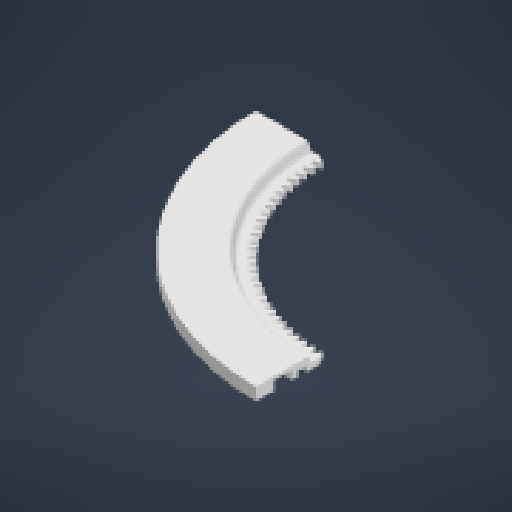
# Autodesk Inventor part: outerspinner_v3
Saved by Autodesk Inventor 2026 (Build 300175050, 175E)
## iProperties
Created: 2026-04-30
Part Number: outerspinner_v3
Material: Generic
Document SubType Name: Modeling
Designer: sniel
Density: 1 g/cm^3
Appearance: Default
Author: sniel
Autodesk Inventor part; units mm, degrees
(part 1 of 2)
ref_plane "YZ Plane" through (0, 0, 0) normal (1, 0, 0) x (0, 1, 0)
ref_plane "XZ Plane" through (0, 0, 0) normal (0, 1, 0) x (-1, 0, 0)
ref_plane "XY Plane" through (0, 0, 0) normal (0, 0, 1) x (1, 0, 0)
sketch "Sketch1" plane through (0, 0, 0) normal (1, 0, 0) x (0, 1, 0)
  line L0 (0, -11.1) -> (7, -11.1)
  line L1 (0, -122.2355) -> (0, -11.1)
  line L2 (13, -122.2355) -> (0, -122.2355)
  line L3 (13, -121.3855) -> (13, -122.2355)
  line L4 (8, -121.3855) -> (13, -121.3855)
  line L5 (8, -115.0855) -> (8, -121.3855)
  line L6 (13, -115.0855) -> (8, -115.0855)
  line L7 (13, -114.2355) -> (13, -115.0855)
  line L8 (7, -114.2355) -> (13, -114.2355)
  line L9 (7, -11.1) -> (7, -114.2355)
  line L10 (7, 11.1) -> (0, 11.1)
  line L11 (7, 114.2355) -> (7, 11.1)
  line L12 (13, 114.2355) -> (7, 114.2355)
  line L13 (13, 115.0855) -> (13, 114.2355)
  line L14 (8, 115.0855) -> (13, 115.0855)
  line L15 (8, 121.3855) -> (8, 115.0855)
  line L16 (13, 121.3855) -> (8, 121.3855)
  line L17 (13, 122.2355) -> (13, 121.3855)
  line L18 (0, 122.2355) -> (13, 122.2355)
  line L19 (0, 11.1) -> (0, 122.2355)
  line L20 (8, 118.2355) -> (13.9, 118.2355)
  line L21 (13.9, 118.2355) -> (13.9, 103.2355)
  line L22 (13.9, 118.2355) -> (13.9, 133.2355)
  line L23 (13.9, 133.2355) -> (15.9, 133.2355)
  line L24 (15.9, 133.2355) -> (15.9, 103.2355)
  line L25 (15.9, 103.2355) -> (13.9, 103.2355)
  line L26 (13.9, 118.2355) -> (13.9, 123.2355)
  line L27 (13.9, 123.2355) -> (8.9, 123.2355)
  line L28 (8.9, 123.2355) -> (8.9, 133.2355)
  line L29 (8.9, 133.2355) -> (13.9, 133.2355)
  line L30 (13.9, 118.2355) -> (13.9, 113.2355)
  line L31 (13.9, 113.2355) -> (8.9, 113.2355)
  line L32 (8.9, 113.2355) -> (8.9, 103.2355)
  line L33 (8.9, 103.2355) -> (13.9, 103.2355)
  line L34 (-3.18, 0) -> (19.08, 0) projected
  dimension "d0" = 5.9
  dimension "d1" = 15
  dimension "d2" = 15
  dimension "d3" = 2
  dimension "d4" = 5
  dimension "d5" = 5
  dimension "d6" = 5
  constraints: 68 end point, 7 perpendicular, 3 horizontal, 2 point on line, 2 vertical, 1 midpoint
  measures "d0" distance of L20.start L20.end
  measures "d1" distance of L20.end L21.end
  measures "d2" distance of L20.end L22.end
  measures "d3" distance of L22.end L23.end
  measures "d4" distance of L20.end L26.end
  measures "d5" distance of L26.end L27.end
  measures "d6" distance of L20.end L30.end
revolve "Revolution1" add sketch "Sketch1" angle 360 about axis through (0, -10, 0) along (0, 1, 0) contours L22 L23 L24 L25 L21 | L21 L33 L32 L31 | L27 L28 L29 L22
sketch "Sketch2" plane through (0, 0, 0) normal (1, 0, 0) x (0, 1, 0)
  line L0 (55, 175) -> (-32, 175)
  line L1 (-32, 175) -> (-32, -166)
  line L2 (-32, -166) -> (55, -166)
  line L3 (55, -166) -> (55, 175)
  point P0 (0, 0)
  constraints: 8 end point, 2 parallel, 1 horizontal, 1 perpendicular
extrude "Extrusion1" cut sketch "Sketch2" along normal blind 157.75
sketch "Sketch3" plane through (0, 8.9, 0) normal (0, -1, 0) x (1, 0, 0)
  arc A0 (-6.4389, -92.6782) -> (-5.913, -96.4432) centre (11.3389, -92.1143) ccw
  arc A1 (-5.913, -96.4432) -> (-4.6085, -96.6498) centre (0, -63.3314) ccw
  arc A2 (-4.6085, -96.6498) -> (-2.9449, -93.2316) centre (-19.6784, -87.2016) ccw
  arc A3 (-2.9449, -93.2316) -> (-1.7688, -93.3241) centre (0, -63.3314) ccw
  arc A4 (-1.7688, -93.3241) -> (-0.6604, -96.9605) centre (15.702, -89.9861) ccw
  arc A5 (-0.6604, -96.9605) -> (0.6604, -96.9605) centre (0, -63.3314) ccw
  arc A6 (0.6604, -96.9605) -> (1.7688, -93.3241) centre (-15.702, -89.9861) ccw
  arc A7 (1.7688, -93.3241) -> (2.9449, -93.2316) centre (0, -63.3314) ccw
  arc A8 (2.9449, -93.2316) -> (4.6085, -96.6498) centre (19.6784, -87.2016) ccw
  arc A9 (4.6085, -96.6498) -> (5.913, -96.4432) centre (0, -63.3314) ccw
  arc A10 (5.913, -96.4432) -> (6.4389, -92.6782) centre (-11.3389, -92.1143) ccw
  arc A11 (6.4389, -92.6782) -> (7.5861, -92.4028) centre (0, -63.3314) ccw
  arc A12 (7.5861, -92.4028) -> (9.7639, -95.5186) centre (23.1702, -83.8294) ccw
  arc A13 (9.7639, -95.5186) -> (11.02, -95.1105) centre (0, -63.3314) ccw
  arc A14 (11.02, -95.1105) -> (10.9505, -91.3096) centre (-6.6967, -93.5337) ccw
  arc A15 (10.9505, -91.3096) -> (12.0404, -90.8581) centre (0, -63.3314) ccw
  arc A16 (12.0404, -90.8581) -> (14.6789, -93.595) centre (26.0915, -79.9524) ccw
  arc A17 (14.6789, -93.595) -> (15.8557, -92.9953) centre (0, -63.3314) ccw
  arc A18 (15.8557, -92.9953) -> (15.1924, -89.2521) centre (-1.8896, -94.2095) ccw
  arc A19 (15.1924, -89.2521) -> (16.1983, -88.6357) centre (0, -63.3314) ccw
  arc A20 (16.1983, -88.6357) -> (19.2324, -90.9261) centre (28.3704, -75.6661) ccw
  arc A21 (19.2324, -90.9261) -> (20.3009, -90.1497) centre (0, -63.3314) ccw
  arc A22 (20.3009, -90.1497) -> (19.0602, -86.5564) centre (2.9641, -94.1249) ccw
  arc A23 (19.0602, -86.5564) -> (19.9574, -85.7902) centre (0, -63.3314) ccw
  arc A24 (19.9574, -85.7902) -> (23.3124, -87.5777) centre (29.9507, -71.0762) ccw
  arc A25 (23.3124, -87.5777) -> (24.2463, -86.6438) centre (0, -63.3314) ccw
  arc A26 (24.2463, -86.6438) -> (22.4588, -83.2888) centre (7.7447, -93.2821) ccw
  arc A27 (22.4588, -83.2888) -> (23.225, -82.3917) centre (0, -63.3314) ccw
  arc A28 (23.225, -82.3917) -> (26.8183, -83.6324) centre (30.7935, -66.2955) ccw
  arc A29 (26.8183, -83.6324) -> (27.5947, -82.5638) centre (0, -63.3314) ccw
  arc A30 (27.5947, -82.5638) -> (25.3043, -79.5297) centre (12.3347, -91.7018) ccw
  arc A31 (25.3043, -79.5297) -> (25.9207, -78.5238) centre (0, -63.3314) ccw
  arc A32 (25.9207, -78.5238) -> (29.6639, -79.1871) centre (30.878, -61.4418) ccw
  arc A33 (29.6639, -79.1871) -> (30.2635, -78.0103) centre (0, -63.3314) ccw
  arc A34 (30.2635, -78.0103) -> (27.5267, -75.3718) centre (16.621, -89.4229) ccw
  arc A35 (27.5267, -75.3718) -> (27.9782, -74.2819) centre (0, -63.3314) ccw
  arc A36 (27.9782, -74.2819) -> (31.7791, -74.3514) centre (30.2023, -56.6347) ccw
  arc A37 (31.7791, -74.3514) -> (32.1872, -73.0953) centre (0, -63.3314) ccw
  arc A38 (32.1872, -73.0953) -> (29.0714, -70.9175) centre (20.4979, -86.5016) ccw
  arc A39 (29.0714, -70.9175) -> (29.3468, -69.7703) centre (0, -63.3314) ccw
  arc A40 (29.3468, -69.7703) -> (33.1117, -69.2444) centre (28.7829, -51.9925) ccw
  arc A41 (33.1117, -69.2444) -> (33.3184, -67.9399) centre (0, -63.3314) ccw
  arc A42 (33.3184, -67.9399) -> (29.9002, -66.2763) centre (23.8702, -83.0098) ccw
  arc A43 (29.9002, -66.2763) -> (29.9927, -65.1002) centre (0, -63.3314) ccw
  arc A44 (29.9927, -65.1002) -> (33.6291, -63.9918) centre (26.6547, -47.6295) ccw
  arc A45 (33.6291, -63.9918) -> (33.6291, -62.671) centre (0, -63.3314) ccw
  arc A46 (33.6291, -62.671) -> (29.9927, -61.5627) centre (26.6547, -79.0334) ccw
  arc A47 (29.9927, -61.5627) -> (29.9002, -60.3865) centre (0, -63.3314) ccw
  arc A48 (29.9002, -60.3865) -> (33.3184, -58.7229) centre (23.8702, -43.6531) ccw
  arc A49 (33.3184, -58.7229) -> (33.1117, -57.4184) centre (0, -63.3314) ccw
  arc A50 (33.1117, -57.4184) -> (29.3468, -56.8925) centre (28.7829, -74.6703) ccw
  arc A51 (29.3468, -56.8925) -> (29.0714, -55.7453) centre (0, -63.3314) ccw
  arc A52 (29.0714, -55.7453) -> (32.1872, -53.5675) centre (20.4979, -40.1612) ccw
  arc A53 (32.1872, -53.5675) -> (31.7791, -52.3114) centre (0, -63.3314) ccw
  arc A54 (31.7791, -52.3114) -> (27.9782, -52.381) centre (30.2023, -70.0281) ccw
  arc A55 (27.9782, -52.381) -> (27.5267, -51.291) centre (0, -63.3314) ccw
  arc A56 (27.5267, -51.291) -> (30.2635, -48.6525) centre (16.621, -37.2399) ccw
  arc A57 (30.2635, -48.6525) -> (29.6639, -47.4757) centre (0, -63.3314) ccw
  arc A58 (29.6639, -47.4757) -> (25.9207, -48.139) centre (30.878, -65.221) ccw
  arc A59 (25.9207, -48.139) -> (25.3043, -47.1331) centre (0, -63.3314) ccw
  arc A60 (25.3043, -47.1331) -> (27.5947, -44.099) centre (12.3347, -34.961) ccw
  arc A61 (27.5947, -44.099) -> (26.8183, -43.0305) centre (0, -63.3314) ccw
  arc A62 (26.8183, -43.0305) -> (23.225, -44.2712) centre (30.7935, -60.3673) ccw
  arc A63 (23.225, -44.2712) -> (22.4588, -43.3741) centre (0, -63.3314) ccw
  arc A64 (22.4588, -43.3741) -> (24.2463, -40.019) centre (7.7447, -33.3807) ccw
  arc A65 (24.2463, -40.019) -> (23.3124, -39.0851) centre (0, -63.3314) ccw
  arc A66 (23.3124, -39.0851) -> (19.9574, -40.8727) centre (29.9507, -55.5867) ccw
  arc A67 (19.9574, -40.8727) -> (19.0602, -40.1064) centre (0, -63.3314) ccw
  arc A68 (19.0602, -40.1064) -> (20.3009, -36.5131) centre (2.9641, -32.5379) ccw
  arc A69 (20.3009, -36.5131) -> (19.2324, -35.7368) centre (0, -63.3314) ccw
  arc A70 (19.2324, -35.7368) -> (16.1983, -38.0271) centre (28.3704, -50.9967) ccw
  arc A71 (16.1983, -38.0271) -> (15.1924, -37.4107) centre (0, -63.3314) ccw
  arc A72 (15.1924, -37.4107) -> (15.8557, -33.6675) centre (-1.8896, -32.4534) ccw
  arc A73 (15.8557, -33.6675) -> (14.6789, -33.0679) centre (0, -63.3314) ccw
  arc A74 (14.6789, -33.0679) -> (12.0404, -35.8047) centre (26.0915, -46.7105) ccw
  arc A75 (12.0404, -35.8047) -> (10.9505, -35.3532) centre (0, -63.3314) ccw
  arc A76 (10.9505, -35.3532) -> (11.02, -31.5523) centre (-6.6967, -33.1291) ccw
  arc A77 (11.02, -31.5523) -> (9.7639, -31.1442) centre (0, -63.3314) ccw
  arc A78 (9.7639, -31.1442) -> (7.5861, -34.2601) centre (23.1702, -42.8335) ccw
  arc A79 (7.5861, -34.2601) -> (6.4389, -33.9846) centre (0, -63.3314) ccw
  arc A80 (6.4389, -33.9846) -> (5.913, -30.2197) centre (-11.3389, -34.5486) ccw
  arc A81 (5.913, -30.2197) -> (4.6085, -30.0131) centre (0, -63.3314) ccw
  arc A82 (4.6085, -30.0131) -> (2.9449, -33.4313) centre (19.6784, -39.4612) ccw
  arc A83 (2.9449, -33.4313) -> (1.7688, -33.3387) centre (0, -63.3314) ccw
  arc A84 (1.7688, -33.3387) -> (0.6604, -29.7023) centre (-15.702, -36.6767) ccw
  arc A85 (0.6604, -29.7023) -> (-0.6604, -29.7023) centre (0, -63.3314) ccw
  arc A86 (-0.6604, -29.7023) -> (-1.7688, -33.3387) centre (15.702, -36.6767) ccw
  arc A87 (-1.7688, -33.3387) -> (-2.9449, -33.4313) centre (0, -63.3314) ccw
  arc A88 (-2.9449, -33.4313) -> (-4.6085, -30.0131) centre (-19.6784, -39.4612) ccw
  arc A89 (-4.6085, -30.0131) -> (-5.913, -30.2197) centre (0, -63.3314) ccw
  arc A90 (-5.913, -30.2197) -> (-6.4389, -33.9846) centre (11.3389, -34.5486) ccw
  arc A91 (-6.4389, -33.9846) -> (-7.5861, -34.2601) centre (0, -63.3314) ccw
  arc A92 (-7.5861, -34.2601) -> (-9.7639, -31.1442) centre (-23.1702, -42.8335) ccw
  arc A93 (-9.7639, -31.1442) -> (-11.02, -31.5523) centre (0, -63.3314) ccw
  arc A94 (-11.02, -31.5523) -> (-10.9505, -35.3532) centre (6.6967, -33.1291) ccw
  arc A95 (-10.9505, -35.3532) -> (-12.0404, -35.8047) centre (0, -63.3314) ccw
  arc A96 (-12.0404, -35.8047) -> (-14.6789, -33.0679) centre (-26.0915, -46.7105) ccw
  arc A97 (-14.6789, -33.0679) -> (-15.8557, -33.6675) centre (0, -63.3314) ccw
  arc A98 (-15.8557, -33.6675) -> (-15.1924, -37.4107) centre (1.8896, -32.4534) ccw
  arc A99 (-15.1924, -37.4107) -> (-16.1983, -38.0271) centre (0, -63.3314) ccw
  arc A100 (-16.1983, -38.0271) -> (-19.2324, -35.7368) centre (-28.3704, -50.9967) ccw
  arc A101 (-19.2324, -35.7368) -> (-20.3009, -36.5131) centre (0, -63.3314) ccw
  arc A102 (-20.3009, -36.5131) -> (-19.0602, -40.1064) centre (-2.9641, -32.5379) ccw
  arc A103 (-19.0602, -40.1064) -> (-19.9574, -40.8727) centre (0, -63.3314) ccw
  arc A104 (-19.9574, -40.8727) -> (-23.3124, -39.0851) centre (-29.9507, -55.5867) ccw
  arc A105 (-23.3124, -39.0851) -> (-24.2463, -40.019) centre (0, -63.3314) ccw
  arc A106 (-24.2463, -40.019) -> (-22.4588, -43.3741) centre (-7.7447, -33.3807) ccw
  arc A107 (-22.4588, -43.3741) -> (-23.225, -44.2712) centre (0, -63.3314) ccw
  arc A108 (-23.225, -44.2712) -> (-26.8183, -43.0305) centre (-30.7935, -60.3673) ccw
  arc A109 (-26.8183, -43.0305) -> (-27.5947, -44.099) centre (0, -63.3314) ccw
  arc A110 (-27.5947, -44.099) -> (-25.3043, -47.1331) centre (-12.3347, -34.961) ccw
  arc A111 (-25.3043, -47.1331) -> (-25.9207, -48.139) centre (0, -63.3314) ccw
  arc A112 (-25.9207, -48.139) -> (-29.6639, -47.4757) centre (-30.878, -65.221) ccw
  arc A113 (-29.6639, -47.4757) -> (-30.2635, -48.6525) centre (0, -63.3314) ccw
  arc A114 (-30.2635, -48.6525) -> (-27.5267, -51.291) centre (-16.621, -37.2399) ccw
  arc A115 (-27.5267, -51.291) -> (-27.9782, -52.381) centre (0, -63.3314) ccw
  arc A116 (-27.9782, -52.381) -> (-31.7791, -52.3114) centre (-30.2023, -70.0281) ccw
  arc A117 (-31.7791, -52.3114) -> (-32.1872, -53.5675) centre (0, -63.3314) ccw
  arc A118 (-32.1872, -53.5675) -> (-29.0714, -55.7453) centre (-20.4979, -40.1612) ccw
  arc A119 (-29.0714, -55.7453) -> (-29.3468, -56.8925) centre (0, -63.3314) ccw
  arc A120 (-29.3468, -56.8925) -> (-33.1117, -57.4184) centre (-28.7829, -74.6703) ccw
  arc A121 (-33.1117, -57.4184) -> (-33.3184, -58.7229) centre (0, -63.3314) ccw
  arc A122 (-33.3184, -58.7229) -> (-29.9002, -60.3865) centre (-23.8702, -43.6531) ccw
  arc A123 (-29.9002, -60.3865) -> (-29.9927, -61.5627) centre (0, -63.3314) ccw
  arc A124 (-29.9927, -61.5627) -> (-33.6291, -62.671) centre (-26.6547, -79.0334) ccw
  arc A125 (-33.6291, -62.671) -> (-33.6291, -63.9918) centre (0, -63.3314) ccw
  arc A126 (-33.6291, -63.9918) -> (-29.9927, -65.1002) centre (-26.6547, -47.6295) ccw
  arc A127 (-29.9927, -65.1002) -> (-29.9002, -66.2763) centre (0, -63.3314) ccw
  arc A128 (-29.9002, -66.2763) -> (-33.3184, -67.9399) centre (-23.8702, -83.0098) ccw
  arc A129 (-33.3184, -67.9399) -> (-33.1117, -69.2444) centre (0, -63.3314) ccw
  arc A130 (-33.1117, -69.2444) -> (-29.3468, -69.7703) centre (-28.7829, -51.9925) ccw
  arc A131 (-29.3468, -69.7703) -> (-29.0714, -70.9175) centre (0, -63.3314) ccw
  arc A132 (-29.0714, -70.9175) -> (-32.1872, -73.0953) centre (-20.4979, -86.5016) ccw
  arc A133 (-32.1872, -73.0953) -> (-31.7791, -74.3514) centre (0, -63.3314) ccw
  arc A134 (-31.7791, -74.3514) -> (-27.9782, -74.2819) centre (-30.2023, -56.6347) ccw
  arc A135 (-27.9782, -74.2819) -> (-27.5267, -75.3718) centre (0, -63.3314) ccw
  arc A136 (-27.5267, -75.3718) -> (-30.2635, -78.0103) centre (-16.621, -89.4229) ccw
  arc A137 (-30.2635, -78.0103) -> (-29.6639, -79.1871) centre (0, -63.3314) ccw
  arc A138 (-29.6639, -79.1871) -> (-25.9207, -78.5238) centre (-30.878, -61.4418) ccw
  arc A139 (-25.9207, -78.5238) -> (-25.3043, -79.5297) centre (0, -63.3314) ccw
  arc A140 (-25.3043, -79.5297) -> (-27.5947, -82.5638) centre (-12.3347, -91.7018) ccw
  arc A141 (-27.5947, -82.5638) -> (-26.8183, -83.6324) centre (0, -63.3314) ccw
  arc A142 (-26.8183, -83.6324) -> (-23.225, -82.3917) centre (-30.7935, -66.2955) ccw
  arc A143 (-23.225, -82.3917) -> (-22.4588, -83.2888) centre (0, -63.3314) ccw
  arc A144 (-22.4588, -83.2888) -> (-24.2463, -86.6438) centre (-7.7447, -93.2821) ccw
  arc A145 (-24.2463, -86.6438) -> (-23.3124, -87.5777) centre (0, -63.3314) ccw
  arc A146 (-23.3124, -87.5777) -> (-19.9574, -85.7902) centre (-29.9507, -71.0762) ccw
  arc A147 (-19.9574, -85.7902) -> (-19.0602, -86.5564) centre (0, -63.3314) ccw
  arc A148 (-19.0602, -86.5564) -> (-20.3009, -90.1497) centre (-2.9641, -94.1249) ccw
  arc A149 (-20.3009, -90.1497) -> (-19.2324, -90.9261) centre (0, -63.3314) ccw
  arc A150 (-19.2324, -90.9261) -> (-16.1983, -88.6357) centre (-28.3704, -75.6661) ccw
  arc A151 (-16.1983, -88.6357) -> (-15.1924, -89.2521) centre (0, -63.3314) ccw
  arc A152 (-15.1924, -89.2521) -> (-15.8557, -92.9953) centre (1.8896, -94.2095) ccw
  arc A153 (-15.8557, -92.9953) -> (-14.6789, -93.595) centre (0, -63.3314) ccw
  arc A154 (-14.6789, -93.595) -> (-12.0404, -90.8581) centre (-26.0915, -79.9524) ccw
  arc A155 (-12.0404, -90.8581) -> (-10.9505, -91.3096) centre (0, -63.3314) ccw
  arc A156 (-10.9505, -91.3096) -> (-11.02, -95.1105) centre (6.6967, -93.5337) ccw
  arc A157 (-11.02, -95.1105) -> (-9.7639, -95.5186) centre (0, -63.3314) ccw
  arc A158 (-9.7639, -95.5186) -> (-7.5861, -92.4028) centre (-23.1702, -83.8294) ccw
  arc A159 (-7.5861, -92.4028) -> (-6.4389, -92.6782) centre (0, -63.3314) ccw
  arc A160 (-6.4389, -29.3468) -> (-5.913, -33.1117) centre (11.3389, -28.7829) ccw
  arc A161 (-5.913, -33.1117) -> (-4.6085, -33.3184) centre (0, 0) ccw
  arc A162 (-4.6085, -33.3184) -> (-2.9449, -29.9002) centre (-19.6784, -23.8702) ccw
  arc A163 (-2.9449, -29.9002) -> (-1.7688, -29.9927) centre (0, 0) ccw
  arc A164 (-1.7688, -29.9927) -> (-0.6604, -33.6291) centre (15.702, -26.6547) ccw
  arc A165 (-0.6604, -33.6291) -> (0.6604, -33.6291) centre (0, 0) ccw
  arc A166 (0.6604, -33.6291) -> (1.7688, -29.9927) centre (-15.702, -26.6547) ccw
  arc A167 (1.7688, -29.9927) -> (2.9449, -29.9002) centre (0, 0) ccw
  arc A168 (2.9449, -29.9002) -> (4.6085, -33.3184) centre (19.6784, -23.8702) ccw
  arc A169 (4.6085, -33.3184) -> (5.913, -33.1117) centre (0, 0) ccw
  arc A170 (5.913, -33.1117) -> (6.4389, -29.3468) centre (-11.3389, -28.7829) ccw
  arc A171 (6.4389, -29.3468) -> (7.5861, -29.0714) centre (0, 0) ccw
  arc A172 (7.5861, -29.0714) -> (9.7639, -32.1872) centre (23.1702, -20.4979) ccw
  arc A173 (9.7639, -32.1872) -> (11.02, -31.7791) centre (0, 0) ccw
  arc A174 (11.02, -31.7791) -> (10.9505, -27.9782) centre (-6.6967, -30.2023) ccw
  arc A175 (10.9505, -27.9782) -> (12.0404, -27.5267) centre (0, 0) ccw
  arc A176 (12.0404, -27.5267) -> (14.6789, -30.2635) centre (26.0915, -16.621) ccw
  arc A177 (14.6789, -30.2635) -> (15.8557, -29.6639) centre (0, 0) ccw
  arc A178 (15.8557, -29.6639) -> (15.1924, -25.9207) centre (-1.8896, -30.878) ccw
  arc A179 (15.1924, -25.9207) -> (16.1983, -25.3043) centre (0, 0) ccw
  arc A180 (16.1983, -25.3043) -> (19.2324, -27.5947) centre (28.3704, -12.3347) ccw
  arc A181 (19.2324, -27.5947) -> (20.3009, -26.8183) centre (0, 0) ccw
  arc A182 (20.3009, -26.8183) -> (19.0602, -23.225) centre (2.9641, -30.7935) ccw
  arc A183 (19.0602, -23.225) -> (19.9574, -22.4588) centre (0, 0) ccw
  arc A184 (19.9574, -22.4588) -> (23.3124, -24.2463) centre (29.9507, -7.7447) ccw
  arc A185 (23.3124, -24.2463) -> (24.2463, -23.3124) centre (0, 0) ccw
  arc A186 (24.2463, -23.3124) -> (22.4588, -19.9574) centre (7.7447, -29.9507) ccw
  arc A187 (22.4588, -19.9574) -> (23.225, -19.0602) centre (0, 0) ccw
  arc A188 (23.225, -19.0602) -> (26.8183, -20.3009) centre (30.7935, -2.9641) ccw
  arc A189 (26.8183, -20.3009) -> (27.5947, -19.2324) centre (0, 0) ccw
  arc A190 (27.5947, -19.2324) -> (25.3043, -16.1983) centre (12.3347, -28.3704) ccw
  arc A191 (25.3043, -16.1983) -> (25.9207, -15.1924) centre (0, 0) ccw
  arc A192 (25.9207, -15.1924) -> (29.6639, -15.8557) centre (30.878, 1.8896) ccw
  arc A193 (29.6639, -15.8557) -> (30.2635, -14.6789) centre (0, 0) ccw
  arc A194 (30.2635, -14.6789) -> (27.5267, -12.0404) centre (16.621, -26.0915) ccw
  arc A195 (27.5267, -12.0404) -> (27.9782, -10.9505) centre (0, 0) ccw
  arc A196 (27.9782, -10.9505) -> (31.7791, -11.02) centre (30.2023, 6.6967) ccw
  arc A197 (31.7791, -11.02) -> (32.1872, -9.7639) centre (0, 0) ccw
  arc A198 (32.1872, -9.7639) -> (29.0714, -7.5861) centre (20.4979, -23.1702) ccw
  arc A199 (29.0714, -7.5861) -> (29.3468, -6.4389) centre (0, 0) ccw
  arc A200 (29.3468, -6.4389) -> (33.1117, -5.913) centre (28.7829, 11.3389) ccw
  arc A201 (33.1117, -5.913) -> (33.3184, -4.6085) centre (0, 0) ccw
  arc A202 (33.3184, -4.6085) -> (29.9002, -2.9449) centre (23.8702, -19.6784) ccw
  arc A203 (29.9002, -2.9449) -> (29.9927, -1.7688) centre (0, 0) ccw
  arc A204 (29.9927, -1.7688) -> (33.6291, -0.6604) centre (26.6547, 15.702) ccw
  arc A205 (33.6291, -0.6604) -> (33.6291, 0.6604) centre (0, 0) ccw
  arc A206 (33.6291, 0.6604) -> (29.9927, 1.7688) centre (26.6547, -15.702) ccw
  arc A207 (29.9927, 1.7688) -> (29.9002, 2.9449) centre (0, 0) ccw
  arc A208 (29.9002, 2.9449) -> (33.3184, 4.6085) centre (23.8702, 19.6784) ccw
  arc A209 (33.3184, 4.6085) -> (33.1117, 5.913) centre (0, 0) ccw
  arc A210 (33.1117, 5.913) -> (29.3468, 6.4389) centre (28.7829, -11.3389) ccw
  arc A211 (29.3468, 6.4389) -> (29.0714, 7.5861) centre (0, 0) ccw
  arc A212 (29.0714, 7.5861) -> (32.1872, 9.7639) centre (20.4979, 23.1702) ccw
  arc A213 (32.1872, 9.7639) -> (31.7791, 11.02) centre (0, 0) ccw
  arc A214 (31.7791, 11.02) -> (27.9782, 10.9505) centre (30.2023, -6.6967) ccw
  arc A215 (27.9782, 10.9505) -> (27.5267, 12.0404) centre (0, 0) ccw
  arc A216 (27.5267, 12.0404) -> (30.2635, 14.6789) centre (16.621, 26.0915) ccw
  arc A217 (30.2635, 14.6789) -> (29.6639, 15.8557) centre (0, 0) ccw
  arc A218 (29.6639, 15.8557) -> (25.9207, 15.1924) centre (30.878, -1.8896) ccw
  arc A219 (25.9207, 15.1924) -> (25.3043, 16.1983) centre (0, 0) ccw
  arc A220 (25.3043, 16.1983) -> (27.5947, 19.2324) centre (12.3347, 28.3704) ccw
  arc A221 (27.5947, 19.2324) -> (26.8183, 20.3009) centre (0, 0) ccw
  arc A222 (26.8183, 20.3009) -> (23.225, 19.0602) centre (30.7935, 2.9641) ccw
  arc A223 (23.225, 19.0602) -> (22.4588, 19.9574) centre (0, 0) ccw
  arc A224 (22.4588, 19.9574) -> (24.2463, 23.3124) centre (7.7447, 29.9507) ccw
  arc A225 (24.2463, 23.3124) -> (23.3124, 24.2463) centre (0, 0) ccw
  arc A226 (23.3124, 24.2463) -> (19.9574, 22.4588) centre (29.9507, 7.7447) ccw
  arc A227 (19.9574, 22.4588) -> (19.0602, 23.225) centre (0, 0) ccw
  arc A228 (19.0602, 23.225) -> (20.3009, 26.8183) centre (2.9641, 30.7935) ccw
  arc A229 (20.3009, 26.8183) -> (19.2324, 27.5947) centre (0, 0) ccw
  arc A230 (19.2324, 27.5947) -> (16.1983, 25.3043) centre (28.3704, 12.3347) ccw
  arc A231 (16.1983, 25.3043) -> (15.1924, 25.9207) centre (0, 0) ccw
  arc A232 (15.1924, 25.9207) -> (15.8557, 29.6639) centre (-1.8896, 30.878) ccw
  arc A233 (15.8557, 29.6639) -> (14.6789, 30.2635) centre (0, 0) ccw
  arc A234 (14.6789, 30.2635) -> (12.0404, 27.5267) centre (26.0915, 16.621) ccw
  arc A235 (12.0404, 27.5267) -> (10.9505, 27.9782) centre (0, 0) ccw
  arc A236 (10.9505, 27.9782) -> (11.02, 31.7791) centre (-6.6967, 30.2023) ccw
  arc A237 (11.02, 31.7791) -> (9.7639, 32.1872) centre (0, 0) ccw
  arc A238 (9.7639, 32.1872) -> (7.5861, 29.0714) centre (23.1702, 20.4979) ccw
  arc A239 (7.5861, 29.0714) -> (6.4389, 29.3468) centre (0, 0) ccw
  arc A240 (6.4389, 29.3468) -> (5.913, 33.1117) centre (-11.3389, 28.7829) ccw
  arc A241 (5.913, 33.1117) -> (4.6085, 33.3184) centre (0, 0) ccw
  arc A242 (4.6085, 33.3184) -> (2.9449, 29.9002) centre (19.6784, 23.8702) ccw
  arc A243 (2.9449, 29.9002) -> (1.7688, 29.9927) centre (0, 0) ccw
  arc A244 (1.7688, 29.9927) -> (0.6604, 33.6291) centre (-15.702, 26.6547) ccw
  arc A245 (0.6604, 33.6291) -> (-0.6604, 33.6291) centre (0, 0) ccw
  arc A246 (-0.6604, 33.6291) -> (-1.7688, 29.9927) centre (15.702, 26.6547) ccw
  arc A247 (-1.7688, 29.9927) -> (-2.9449, 29.9002) centre (0, 0) ccw
  arc A248 (-2.9449, 29.9002) -> (-4.6085, 33.3184) centre (-19.6784, 23.8702) ccw
  arc A249 (-4.6085, 33.3184) -> (-5.913, 33.1117) centre (0, 0) ccw
  arc A250 (-5.913, 33.1117) -> (-6.4389, 29.3468) centre (11.3389, 28.7829) ccw
  arc A251 (-6.4389, 29.3468) -> (-7.5861, 29.0714) centre (0, 0) ccw
  arc A252 (-7.5861, 29.0714) -> (-9.7639, 32.1872) centre (-23.1702, 20.4979) ccw
  arc A253 (-9.7639, 32.1872) -> (-11.02, 31.7791) centre (0, 0) ccw
  arc A254 (-11.02, 31.7791) -> (-10.9505, 27.9782) centre (6.6967, 30.2023) ccw
  arc A255 (-10.9505, 27.9782) -> (-12.0404, 27.5267) centre (0, 0) ccw
  arc A256 (-12.0404, 27.5267) -> (-14.6789, 30.2635) centre (-26.0915, 16.621) ccw
  arc A257 (-14.6789, 30.2635) -> (-15.8557, 29.6639) centre (0, 0) ccw
  arc A258 (-15.8557, 29.6639) -> (-15.1924, 25.9207) centre (1.8896, 30.878) ccw
  arc A259 (-15.1924, 25.9207) -> (-16.1983, 25.3043) centre (0, 0) ccw
  arc A260 (-16.1983, 25.3043) -> (-19.2324, 27.5947) centre (-28.3704, 12.3347) ccw
  arc A261 (-19.2324, 27.5947) -> (-20.3009, 26.8183) centre (0, 0) ccw
  arc A262 (-20.3009, 26.8183) -> (-19.0602, 23.225) centre (-2.9641, 30.7935) ccw
  arc A263 (-19.0602, 23.225) -> (-19.9574, 22.4588) centre (0, 0) ccw
  arc A264 (-19.9574, 22.4588) -> (-23.3124, 24.2463) centre (-29.9507, 7.7447) ccw
  arc A265 (-23.3124, 24.2463) -> (-24.2463, 23.3124) centre (0, 0) ccw
  arc A266 (-24.2463, 23.3124) -> (-22.4588, 19.9574) centre (-7.7447, 29.9507) ccw
  arc A267 (-22.4588, 19.9574) -> (-23.225, 19.0602) centre (0, 0) ccw
  arc A268 (-23.225, 19.0602) -> (-26.8183, 20.3009) centre (-30.7935, 2.9641) ccw
  arc A269 (-26.8183, 20.3009) -> (-27.5947, 19.2324) centre (0, 0) ccw
  arc A270 (-27.5947, 19.2324) -> (-25.3043, 16.1983) centre (-12.3347, 28.3704) ccw
  arc A271 (-25.3043, 16.1983) -> (-25.9207, 15.1924) centre (0, 0) ccw
  arc A272 (-25.9207, 15.1924) -> (-29.6639, 15.8557) centre (-30.878, -1.8896) ccw
  arc A273 (-29.6639, 15.8557) -> (-30.2635, 14.6789) centre (0, 0) ccw
  arc A274 (-30.2635, 14.6789) -> (-27.5267, 12.0404) centre (-16.621, 26.0915) ccw
  arc A275 (-27.5267, 12.0404) -> (-27.9782, 10.9505) centre (0, 0) ccw
  arc A276 (-27.9782, 10.9505) -> (-31.7791, 11.02) centre (-30.2023, -6.6967) ccw
  arc A277 (-31.7791, 11.02) -> (-32.1872, 9.7639) centre (0, 0) ccw
  arc A278 (-32.1872, 9.7639) -> (-29.0714, 7.5861) centre (-20.4979, 23.1702) ccw
  arc A279 (-29.0714, 7.5861) -> (-29.3468, 6.4389) centre (0, 0) ccw
  arc A280 (-29.3468, 6.4389) -> (-33.1117, 5.913) centre (-28.7829, -11.3389) ccw
  arc A281 (-33.1117, 5.913) -> (-33.3184, 4.6085) centre (0, 0) ccw
  arc A282 (-33.3184, 4.6085) -> (-29.9002, 2.9449) centre (-23.8702, 19.6784) ccw
  arc A283 (-29.9002, 2.9449) -> (-29.9927, 1.7688) centre (0, 0) ccw
  arc A284 (-29.9927, 1.7688) -> (-33.6291, 0.6604) centre (-26.6547, -15.702) ccw
  arc A285 (-33.6291, 0.6604) -> (-33.6291, -0.6604) centre (0, 0) ccw
  arc A286 (-33.6291, -0.6604) -> (-29.9927, -1.7688) centre (-26.6547, 15.702) ccw
  arc A287 (-29.9927, -1.7688) -> (-29.9002, -2.9449) centre (0, 0) ccw
  arc A288 (-29.9002, -2.9449) -> (-33.3184, -4.6085) centre (-23.8702, -19.6784) ccw
  arc A289 (-33.3184, -4.6085) -> (-33.1117, -5.913) centre (0, 0) ccw
  arc A290 (-33.1117, -5.913) -> (-29.3468, -6.4389) centre (-28.7829, 11.3389) ccw
  arc A291 (-29.3468, -6.4389) -> (-29.0714, -7.5861) centre (0, 0) ccw
  arc A292 (-29.0714, -7.5861) -> (-32.1872, -9.7639) centre (-20.4979, -23.1702) ccw
  arc A293 (-32.1872, -9.7639) -> (-31.7791, -11.02) centre (0, 0) ccw
  arc A294 (-31.7791, -11.02) -> (-27.9782, -10.9505) centre (-30.2023, 6.6967) ccw
  arc A295 (-27.9782, -10.9505) -> (-27.5267, -12.0404) centre (0, 0) ccw
  arc A296 (-27.5267, -12.0404) -> (-30.2635, -14.6789) centre (-16.621, -26.0915) ccw
  arc A297 (-30.2635, -14.6789) -> (-29.6639, -15.8557) centre (0, 0) ccw
  arc A298 (-29.6639, -15.8557) -> (-25.9207, -15.1924) centre (-30.878, 1.8896) ccw
  arc A299 (-25.9207, -15.1924) -> (-25.3043, -16.1983) centre (0, 0) ccw
  arc A300 (-25.3043, -16.1983) -> (-27.5947, -19.2324) centre (-12.3347, -28.3704) ccw
  arc A301 (-27.5947, -19.2324) -> (-26.8183, -20.3009) centre (0, 0) ccw
  arc A302 (-26.8183, -20.3009) -> (-23.225, -19.0602) centre (-30.7935, -2.9641) ccw
  arc A303 (-23.225, -19.0602) -> (-22.4588, -19.9574) centre (0, 0) ccw
  arc A304 (-22.4588, -19.9574) -> (-24.2463, -23.3124) centre (-7.7447, -29.9507) ccw
  arc A305 (-24.2463, -23.3124) -> (-23.3124, -24.2463) centre (0, 0) ccw
  arc A306 (-23.3124, -24.2463) -> (-19.9574, -22.4588) centre (-29.9507, -7.7447) ccw
  arc A307 (-19.9574, -22.4588) -> (-19.0602, -23.225) centre (0, 0) ccw
  arc A308 (-19.0602, -23.225) -> (-20.3009, -26.8183) centre (-2.9641, -30.7935) ccw
  arc A309 (-20.3009, -26.8183) -> (-19.2324, -27.5947) centre (0, 0) ccw
  arc A310 (-19.2324, -27.5947) -> (-16.1983, -25.3043) centre (-28.3704, -12.3347) ccw
  arc A311 (-16.1983, -25.3043) -> (-15.1924, -25.9207) centre (0, 0) ccw
  arc A312 (-15.1924, -25.9207) -> (-15.8557, -29.6639) centre (1.8896, -30.878) ccw
  arc A313 (-15.8557, -29.6639) -> (-14.6789, -30.2635) centre (0, 0) ccw
  arc A314 (-14.6789, -30.2635) -> (-12.0404, -27.5267) centre (-26.0915, -16.621) ccw
  arc A315 (-12.0404, -27.5267) -> (-10.9505, -27.9782) centre (0, 0) ccw
  arc A316 (-10.9505, -27.9782) -> (-11.02, -31.7791) centre (6.6967, -30.2023) ccw
  arc A317 (-11.02, -31.7791) -> (-9.7639, -32.1872) centre (0, 0) ccw
  arc A318 (-9.7639, -32.1872) -> (-7.5861, -29.0714) centre (-23.1702, -20.4979) ccw
  arc A319 (-7.5861, -29.0714) -> (-6.4389, -29.3468) centre (0, 0) ccw
  arc A320 (-6.7466, -93.5477) -> (-5.7329, -97.2125) centre (16.0081, -89.2263) ccw
  arc A321 (-7.9705, -93.4514) -> (-6.7466, -93.5477) centre (0, 0) ccw
  arc A322 (-9.545, -96.9125) -> (-7.9705, -93.4514) centre (-29.769, -85.6236) ccw
  arc A323 (-10.8128, -96.7792) -> (-9.545, -96.9125) centre (0, 0) ccw
  arc A324 (-11.6333, -93.0664) -> (-10.8128, -96.7792) centre (11.3164, -89.9418) ccw
  arc A325 (-12.8505, -92.9062) -> (-11.6333, -93.0664) centre (0, 0) ccw
  arc A326 (-14.604, -96.2801) -> (-12.8505, -92.9062) centre (-34.2094, -83.9482) ccw
  arc A327 (-15.863, -96.0807) -> (-14.604, -96.2801) centre (0, 0) ccw
  arc A328 (-16.4881, -92.33) -> (-15.863, -96.0807) centre (6.5937, -90.4108) ccw
  arc A329 (-17.6952, -92.1063) -> (-16.4881, -92.33) centre (0, 0) ccw
  arc A330 (-19.6229, -95.3839) -> (-17.6952, -92.1063) centre (-38.5561, -82.0428) ccw
  arc A331 (-20.8697, -95.1188) -> (-19.6229, -95.3839) centre (0, 0) ccw
  arc A332 (-21.2976, -91.3406) -> (-20.8697, -95.1188) centre (1.8529, -90.632) ccw
  arc A333 (-22.4914, -91.054) -> (-21.2976, -91.3406) centre (0, 0) ccw
  arc A334 (-24.588, -94.2261) -> (-22.4914, -91.054) centre (-42.797, -79.9125) ccw
  arc A335 (-25.8193, -93.8962) -> (-24.588, -94.2261) centre (0, 0) ccw
  arc A336 (-26.0488, -90.1008) -> (-25.8193, -93.8962) centre (-2.8929, -90.6048) ccw
  arc A337 (-27.226, -89.7521) -> (-26.0488, -90.1008) centre (0, 0) ccw
  arc A338 (-29.4857, -92.8102) -> (-27.226, -89.7521) centre (-46.9207, -77.5632) ccw
  arc A339 (-30.698, -92.4163) -> (-29.4857, -92.8102) centre (0, 0) ccw
  arc A340 (-30.7287, -88.614) -> (-30.698, -92.4163) centre (-7.6309, -90.3292) ccw
  arc A341 (-31.8859, -88.2042) -> (-30.7287, -88.614) centre (0, 0) ccw
  arc A342 (-34.3026, -91.1398) -> (-31.8859, -88.2042) centre (-50.9157, -75.0012) ccw
  arc A343 (-35.4926, -90.683) -> (-34.3026, -91.1398) centre (0, 0) ccw
  arc A344 (-35.3242, -86.8843) -> (-35.4926, -90.683) centre (-12.3479, -89.806) ccw
  arc A345 (-36.4585, -86.4145) -> (-35.3242, -86.8843) centre (0, 0) ccw
  arc A346 (-39.0255, -89.2197) -> (-36.4585, -86.4145) centre (-54.7712, -72.2337) ccw
  arc A347 (-40.19, -88.7012) -> (-39.0255, -89.2197) centre (0, 0) ccw
  arc A348 (-39.823, -84.9165) -> (-40.19, -88.7012) centre (-17.031, -89.0367) ccw
  arc A349 (-40.9311, -84.388) -> (-39.823, -84.9165) centre (0, 0) ccw
  arc A350 (-43.6414, -87.055) -> (-40.9311, -84.388) centre (-58.4765, -69.2682) ccw
  arc A351 (-44.7772, -86.4762) -> (-43.6414, -87.055) centre (0, 0) ccw
  arc A352 (-44.2126, -82.716) -> (-44.7772, -86.4762) centre (-21.6675, -88.0234) ccw
  arc A353 (-45.2915, -82.1302) -> (-44.2126, -82.716) centre (0, 0) ccw
  arc A354 (-48.1377, -84.6516) -> (-45.2915, -82.1302) centre (-62.0216, -66.1129) ccw
  arc A355 (-49.2416, -84.0143) -> (-48.1377, -84.6516) centre (0, 0) ccw
  arc A356 (-48.481, -80.2887) -> (-49.2416, -84.0143) centre (-26.2446, -86.7687) ccw
  arc A357 (-49.5278, -79.6472) -> (-48.481, -80.2887) centre (0, 0) ccw
  arc A358 (-52.502, -82.0163) -> (-49.5278, -79.6472) centre (-65.3967, -62.7763) ccw
  arc A359 (-53.5711, -81.322) -> (-52.502, -82.0163) centre (0, 0) ccw
  arc A360 (-52.6166, -77.6414) -> (-53.5711, -81.322) centre (-30.7498, -85.2763) ccw
  arc A361 (-53.6284, -76.946) -> (-52.6166, -77.6414) centre (0, 0) ccw
  arc A362 (-56.7225, -79.1561) -> (-53.6284, -76.946) centre (-68.5925, -59.2677) ccw
  arc A363 (-57.7538, -78.4069) -> (-56.7225, -79.1561) centre (0, 0) ccw
  arc A364 (-56.6079, -74.7812) -> (-57.7538, -78.4069) centre (-35.1706, -83.5501) ccw
  arc A365 (-57.5819, -74.0339) -> (-56.6079, -74.7812) centre (0, 0) ccw
  arc A366 (-60.7875, -76.079) -> (-57.5819, -74.0339) centre (-71.6004, -55.5966) ccw
  arc A367 (-61.7781, -75.2768) -> (-60.7875, -76.079) centre (0, 0) ccw
  arc A368 (-60.4441, -71.7161) -> (-61.7781, -75.2768) centre (-39.4951, -81.5949) ccw
  arc A369 (-61.3776, -70.9188) -> (-60.4441, -71.7161) centre (0, 0) ccw
  arc A370 (-64.6858, -72.7934) -> (-61.3776, -70.9188) centre (-74.4119, -51.7731) ccw
  arc A371 (-65.6331, -71.9405) -> (-64.6858, -72.7934) centre (0, 0) ccw
  arc A372 (-64.1146, -68.4544) -> (-65.6331, -71.9405) centre (-43.7113, -79.4161) ccw
  arc A373 (-65.0051, -67.6093) -> (-64.1146, -68.4544) centre (0, 0) ccw
  arc A374 (-68.4069, -69.3082) -> (-65.0051, -67.6093) centre (-77.0195, -47.8077) ccw
  arc A375 (-69.3082, -68.4069) -> (-68.4069, -69.3082) centre (0, 0) ccw
  arc A376 (-67.6093, -65.0051) -> (-69.3082, -68.4069) centre (-47.8077, -77.0195) ccw
  arc A377 (-68.4544, -64.1146) -> (-67.6093, -65.0051) centre (0, 0) ccw
  arc A378 (-71.9405, -65.6331) -> (-68.4544, -64.1146) centre (-79.4161, -43.7113) ccw
  arc A379 (-72.7934, -64.6858) -> (-71.9405, -65.6331) centre (0, 0) ccw
  arc A380 (-70.9188, -61.3776) -> (-72.7934, -64.6858) centre (-51.7731, -74.4119) ccw
  arc A381 (-71.7161, -60.4441) -> (-70.9188, -61.3776) centre (0, 0) ccw
  arc A382 (-75.2768, -61.7781) -> (-71.7161, -60.4441) centre (-81.5949, -39.4951) ccw
  arc A383 (-76.079, -60.7875) -> (-75.2768, -61.7781) centre (0, 0) ccw
  arc A384 (-74.0339, -57.5819) -> (-76.079, -60.7875) centre (-55.5966, -71.6004) ccw
  arc A385 (-74.7812, -56.6079) -> (-74.0339, -57.5819) centre (0, 0) ccw
  arc A386 (-78.4069, -57.7538) -> (-74.7812, -56.6079) centre (-83.5501, -35.1706) ccw
  arc A387 (-79.1561, -56.7225) -> (-78.4069, -57.7538) centre (0, 0) ccw
  arc A388 (-76.946, -53.6284) -> (-79.1561, -56.7225) centre (-59.2677, -68.5925) ccw
  arc A389 (-77.6414, -52.6166) -> (-76.946, -53.6284) centre (0, 0) ccw
  arc A390 (-81.322, -53.5711) -> (-77.6414, -52.6166) centre (-85.2763, -30.7498) ccw
  arc A391 (-82.0163, -52.502) -> (-81.322, -53.5711) centre (0, 0) ccw
  arc A392 (-79.6472, -49.5278) -> (-82.0163, -52.502) centre (-62.7763, -65.3967) ccw
  arc A393 (-80.2887, -48.481) -> (-79.6472, -49.5278) centre (0, 0) ccw
  arc A394 (-84.0143, -49.2416) -> (-80.2887, -48.481) centre (-86.7687, -26.2446) ccw
  arc A395 (-84.6516, -48.1377) -> (-84.0143, -49.2416) centre (0, 0) ccw
  arc A396 (-82.1302, -45.2915) -> (-84.6516, -48.1377) centre (-66.1129, -62.0216) ccw
  arc A397 (-82.716, -44.2126) -> (-82.1302, -45.2915) centre (0, 0) ccw
  arc A398 (-86.4762, -44.7772) -> (-82.716, -44.2126) centre (-88.0234, -21.6675) ccw
  arc A399 (-87.055, -43.6414) -> (-86.4762, -44.7772) centre (0, 0) ccw
  arc A400 (-84.388, -40.9311) -> (-87.055, -43.6414) centre (-69.2682, -58.4765) ccw
  arc A401 (-84.9165, -39.823) -> (-84.388, -40.9311) centre (0, 0) ccw
  arc A402 (-88.7012, -40.19) -> (-84.9165, -39.823) centre (-89.0367, -17.031) ccw
  arc A403 (-89.2197, -39.0255) -> (-88.7012, -40.19) centre (0, 0) ccw
  arc A404 (-86.4145, -36.4585) -> (-89.2197, -39.0255) centre (-72.2337, -54.7712) ccw
  arc A405 (-86.8843, -35.3242) -> (-86.4145, -36.4585) centre (0, 0) ccw
  arc A406 (-90.683, -35.4926) -> (-86.8843, -35.3242) centre (-89.806, -12.3479) ccw
  arc A407 (-91.1398, -34.3026) -> (-90.683, -35.4926) centre (0, 0) ccw
  arc A408 (-88.2042, -31.8859) -> (-91.1398, -34.3026) centre (-75.0012, -50.9157) ccw
  arc A409 (-88.614, -30.7287) -> (-88.2042, -31.8859) centre (0, 0) ccw
  arc A410 (-92.4163, -30.698) -> (-88.614, -30.7287) centre (-90.3292, -7.6309) ccw
  arc A411 (-92.8102, -29.4857) -> (-92.4163, -30.698) centre (0, 0) ccw
  arc A412 (-89.7521, -27.226) -> (-92.8102, -29.4857) centre (-77.5632, -46.9207) ccw
  arc A413 (-90.1008, -26.0488) -> (-89.7521, -27.226) centre (0, 0) ccw
  arc A414 (-93.8962, -25.8193) -> (-90.1008, -26.0488) centre (-90.6048, -2.8929) ccw
  arc A415 (-94.2261, -24.588) -> (-93.8962, -25.8193) centre (0, 0) ccw
  arc A416 (-91.054, -22.4914) -> (-94.2261, -24.588) centre (-79.9125, -42.797) ccw
  arc A417 (-91.3406, -21.2976) -> (-91.054, -22.4914) centre (0, 0) ccw
  arc A418 (-95.1188, -20.8697) -> (-91.3406, -21.2976) centre (-90.632, 1.8529) ccw
  arc A419 (-95.3839, -19.6229) -> (-95.1188, -20.8697) centre (0, 0) ccw
  arc A420 (-92.1063, -17.6952) -> (-95.3839, -19.6229) centre (-82.0428, -38.5561) ccw
  arc A421 (-92.33, -16.4881) -> (-92.1063, -17.6952) centre (0, 0) ccw
  arc A422 (-96.0807, -15.863) -> (-92.33, -16.4881) centre (-90.4108, 6.5937) ccw
  arc A423 (-96.2801, -14.604) -> (-96.0807, -15.863) centre (0, 0) ccw
  arc A424 (-92.9062, -12.8505) -> (-96.2801, -14.604) centre (-83.9482, -34.2094) ccw
  arc A425 (-93.0664, -11.6333) -> (-92.9062, -12.8505) centre (0, 0) ccw
  arc A426 (-96.7792, -10.8128) -> (-93.0664, -11.6333) centre (-89.9418, 11.3164) ccw
  arc A427 (-96.9125, -9.545) -> (-96.7792, -10.8128) centre (0, 0) ccw
  arc A428 (-93.4514, -7.9705) -> (-96.9125, -9.545) centre (-85.6236, -29.769) ccw
  arc A429 (-93.5477, -6.7466) -> (-93.4514, -7.9705) centre (0, 0) ccw
  arc A430 (-97.2125, -5.7329) -> (-93.5477, -6.7466) centre (-89.2263, 16.0081) ccw
  arc A431 (-97.2792, -4.46) -> (-97.2125, -5.7329) centre (0, 0) ccw
  arc A432 (-93.7404, -3.0687) -> (-97.2792, -4.46) centre (-87.0642, -25.2471) ccw
  arc A433 (-93.7726, -1.8415) -> (-93.7404, -3.0687) centre (0, 0) ccw
  arc A434 (-97.3793, -0.6374) -> (-93.7726, -1.8415) centre (-88.2662, 20.6559) ccw
  arc A435 (-97.3793, 0.6374) -> (-97.3793, -0.6374) centre (0, 0) ccw
  arc A436 (-93.7726, 1.8415) -> (-97.3793, 0.6374) centre (-88.2662, -20.6559) ccw
  arc A437 (-93.7404, 3.0687) -> (-93.7726, 1.8415) centre (0, 0) ccw
  arc A438 (-97.2792, 4.46) -> (-93.7404, 3.0687) centre (-87.0642, 25.2471) ccw
  arc A439 (-97.2125, 5.7329) -> (-97.2792, 4.46) centre (0, 0) ccw
  arc A440 (-93.5477, 6.7466) -> (-97.2125, 5.7329) centre (-89.2263, -16.0081) ccw
  arc A441 (-93.4514, 7.9705) -> (-93.5477, 6.7466) centre (0, 0) ccw
  arc A442 (-96.9125, 9.545) -> (-93.4514, 7.9705) centre (-85.6236, 29.769) ccw
  arc A443 (-96.7792, 10.8128) -> (-96.9125, 9.545) centre (0, 0) ccw
  arc A444 (-93.0664, 11.6333) -> (-96.7792, 10.8128) centre (-89.9418, -11.3164) ccw
  arc A445 (-92.9062, 12.8505) -> (-93.0664, 11.6333) centre (0, 0) ccw
  arc A446 (-96.2801, 14.604) -> (-92.9062, 12.8505) centre (-83.9482, 34.2094) ccw
  arc A447 (-96.0807, 15.863) -> (-96.2801, 14.604) centre (0, 0) ccw
  arc A448 (-92.33, 16.4881) -> (-96.0807, 15.863) centre (-90.4108, -6.5937) ccw
  arc A449 (-92.1063, 17.6952) -> (-92.33, 16.4881) centre (0, 0) ccw
  arc A450 (-95.3839, 19.6229) -> (-92.1063, 17.6952) centre (-82.0428, 38.5561) ccw
  arc A451 (-95.1188, 20.8697) -> (-95.3839, 19.6229) centre (0, 0) ccw
  arc A452 (-91.3406, 21.2976) -> (-95.1188, 20.8697) centre (-90.632, -1.8529) ccw
  arc A453 (-91.054, 22.4914) -> (-91.3406, 21.2976) centre (0, 0) ccw
  arc A454 (-94.2261, 24.588) -> (-91.054, 22.4914) centre (-79.9125, 42.797) ccw
  arc A455 (-93.8962, 25.8193) -> (-94.2261, 24.588) centre (0, 0) ccw
  arc A456 (-90.1008, 26.0488) -> (-93.8962, 25.8193) centre (-90.6048, 2.8929) ccw
  arc A457 (-89.7521, 27.226) -> (-90.1008, 26.0488) centre (0, 0) ccw
  arc A458 (-92.8102, 29.4857) -> (-89.7521, 27.226) centre (-77.5632, 46.9207) ccw
  arc A459 (-92.4163, 30.698) -> (-92.8102, 29.4857) centre (0, 0) ccw
  arc A460 (-88.614, 30.7287) -> (-92.4163, 30.698) centre (-90.3292, 7.6309) ccw
  arc A461 (-88.2042, 31.8859) -> (-88.614, 30.7287) centre (0, 0) ccw
  arc A462 (-91.1398, 34.3026) -> (-88.2042, 31.8859) centre (-75.0012, 50.9157) ccw
  arc A463 (-90.683, 35.4926) -> (-91.1398, 34.3026) centre (0, 0) ccw
  arc A464 (-86.8843, 35.3242) -> (-90.683, 35.4926) centre (-89.806, 12.3479) ccw
  arc A465 (-86.4145, 36.4585) -> (-86.8843, 35.3242) centre (0, 0) ccw
  arc A466 (-89.2197, 39.0255) -> (-86.4145, 36.4585) centre (-72.2337, 54.7712) ccw
  arc A467 (-88.7012, 40.19) -> (-89.2197, 39.0255) centre (0, 0) ccw
  arc A468 (-84.9165, 39.823) -> (-88.7012, 40.19) centre (-89.0367, 17.031) ccw
  arc A469 (-84.388, 40.9311) -> (-84.9165, 39.823) centre (0, 0) ccw
  arc A470 (-87.055, 43.6414) -> (-84.388, 40.9311) centre (-69.2682, 58.4765) ccw
  arc A471 (-86.4762, 44.7772) -> (-87.055, 43.6414) centre (0, 0) ccw
  arc A472 (-82.716, 44.2126) -> (-86.4762, 44.7772) centre (-88.0234, 21.6675) ccw
  arc A473 (-82.1302, 45.2915) -> (-82.716, 44.2126) centre (0, 0) ccw
  arc A474 (-84.6516, 48.1377) -> (-82.1302, 45.2915) centre (-66.1129, 62.0216) ccw
  arc A475 (-84.0143, 49.2416) -> (-84.6516, 48.1377) centre (0, 0) ccw
  arc A476 (-80.2887, 48.481) -> (-84.0143, 49.2416) centre (-86.7687, 26.2446) ccw
  arc A477 (-79.6472, 49.5278) -> (-80.2887, 48.481) centre (0, 0) ccw
  arc A478 (-82.0163, 52.502) -> (-79.6472, 49.5278) centre (-62.7763, 65.3967) ccw
  arc A479 (-81.322, 53.5711) -> (-82.0163, 52.502) centre (0, 0) ccw
  arc A480 (-77.6414, 52.6166) -> (-81.322, 53.5711) centre (-85.2763, 30.7498) ccw
  arc A481 (-76.946, 53.6284) -> (-77.6414, 52.6166) centre (0, 0) ccw
  arc A482 (-79.1561, 56.7225) -> (-76.946, 53.6284) centre (-59.2677, 68.5925) ccw
  arc A483 (-78.4069, 57.7538) -> (-79.1561, 56.7225) centre (0, 0) ccw
  arc A484 (-74.7812, 56.6079) -> (-78.4069, 57.7538) centre (-83.5501, 35.1706) ccw
  arc A485 (-74.0339, 57.5819) -> (-74.7812, 56.6079) centre (0, 0) ccw
  arc A486 (-76.079, 60.7875) -> (-74.0339, 57.5819) centre (-55.5966, 71.6004) ccw
  arc A487 (-75.2768, 61.7781) -> (-76.079, 60.7875) centre (0, 0) ccw
  arc A488 (-71.7161, 60.4441) -> (-75.2768, 61.7781) centre (-81.5949, 39.4951) ccw
  arc A489 (-70.9188, 61.3776) -> (-71.7161, 60.4441) centre (0, 0) ccw
  arc A490 (-72.7934, 64.6858) -> (-70.9188, 61.3776) centre (-51.7731, 74.4119) ccw
  arc A491 (-71.9405, 65.6331) -> (-72.7934, 64.6858) centre (0, 0) ccw
  arc A492 (-68.4544, 64.1146) -> (-71.9405, 65.6331) centre (-79.4161, 43.7113) ccw
  arc A493 (-67.6093, 65.0051) -> (-68.4544, 64.1146) centre (0, 0) ccw
  arc A494 (-69.3082, 68.4069) -> (-67.6093, 65.0051) centre (-47.8077, 77.0195) ccw
  arc A495 (-68.4069, 69.3082) -> (-69.3082, 68.4069) centre (0, 0) ccw
  arc A496 (-65.0051, 67.6093) -> (-68.4069, 69.3082) centre (-77.0195, 47.8077) ccw
  arc A497 (-64.1146, 68.4544) -> (-65.0051, 67.6093) centre (0, 0) ccw
  arc A498 (-65.6331, 71.9405) -> (-64.1146, 68.4544) centre (-43.7113, 79.4161) ccw
  arc A499 (-64.6858, 72.7934) -> (-65.6331, 71.9405) centre (0, 0) ccw
  arc A500 (-61.3776, 70.9188) -> (-64.6858, 72.7934) centre (-74.4119, 51.7731) ccw
  arc A501 (-60.4441, 71.7161) -> (-61.3776, 70.9188) centre (0, 0) ccw
  arc A502 (-61.7781, 75.2768) -> (-60.4441, 71.7161) centre (-39.4951, 81.5949) ccw
  arc A503 (-60.7875, 76.079) -> (-61.7781, 75.2768) centre (0, 0) ccw
  arc A504 (-57.5819, 74.0339) -> (-60.7875, 76.079) centre (-71.6004, 55.5966) ccw
  arc A505 (-56.6079, 74.7812) -> (-57.5819, 74.0339) centre (0, 0) ccw
  arc A506 (-57.7538, 78.4069) -> (-56.6079, 74.7812) centre (-35.1706, 83.5501) ccw
  arc A507 (-56.7225, 79.1561) -> (-57.7538, 78.4069) centre (0, 0) ccw
  arc A508 (-53.6284, 76.946) -> (-56.7225, 79.1561) centre (-68.5925, 59.2677) ccw
  arc A509 (-52.6166, 77.6414) -> (-53.6284, 76.946) centre (0, 0) ccw
  arc A510 (-53.5711, 81.322) -> (-52.6166, 77.6414) centre (-30.7498, 85.2763) ccw
  arc A511 (-52.502, 82.0163) -> (-53.5711, 81.322) centre (0, 0) ccw
  arc A512 (-49.5278, 79.6472) -> (-52.502, 82.0163) centre (-65.3967, 62.7763) ccw
  arc A513 (-48.481, 80.2887) -> (-49.5278, 79.6472) centre (0, 0) ccw
  arc A514 (-49.2416, 84.0143) -> (-48.481, 80.2887) centre (-26.2446, 86.7687) ccw
  arc A515 (-48.1377, 84.6516) -> (-49.2416, 84.0143) centre (0, 0) ccw
  arc A516 (-45.2915, 82.1302) -> (-48.1377, 84.6516) centre (-62.0216, 66.1129) ccw
  arc A517 (-44.2126, 82.716) -> (-45.2915, 82.1302) centre (0, 0) ccw
  arc A518 (-44.7772, 86.4762) -> (-44.2126, 82.716) centre (-21.6675, 88.0234) ccw
  arc A519 (-43.6414, 87.055) -> (-44.7772, 86.4762) centre (0, 0) ccw
  arc A520 (-40.9311, 84.388) -> (-43.6414, 87.055) centre (-58.4765, 69.2682) ccw
  arc A521 (-39.823, 84.9165) -> (-40.9311, 84.388) centre (0, 0) ccw
  arc A522 (-40.19, 88.7012) -> (-39.823, 84.9165) centre (-17.031, 89.0367) ccw
  arc A523 (-39.0255, 89.2197) -> (-40.19, 88.7012) centre (0, 0) ccw
  arc A524 (-36.4585, 86.4145) -> (-39.0255, 89.2197) centre (-54.7712, 72.2337) ccw
  arc A525 (-35.3242, 86.8843) -> (-36.4585, 86.4145) centre (0, 0) ccw
  arc A526 (-35.4926, 90.683) -> (-35.3242, 86.8843) centre (-12.3479, 89.806) ccw
  arc A527 (-34.3026, 91.1398) -> (-35.4926, 90.683) centre (0, 0) ccw
  arc A528 (-31.8859, 88.2042) -> (-34.3026, 91.1398) centre (-50.9157, 75.0012) ccw
  arc A529 (-30.7287, 88.614) -> (-31.8859, 88.2042) centre (0, 0) ccw
  arc A530 (-30.698, 92.4163) -> (-30.7287, 88.614) centre (-7.6309, 90.3292) ccw
  arc A531 (-29.4857, 92.8102) -> (-30.698, 92.4163) centre (0, 0) ccw
  arc A532 (-27.226, 89.7521) -> (-29.4857, 92.8102) centre (-46.9207, 77.5632) ccw
  arc A533 (-26.0488, 90.1008) -> (-27.226, 89.7521) centre (0, 0) ccw
  arc A534 (-25.8193, 93.8962) -> (-26.0488, 90.1008) centre (-2.8929, 90.6048) ccw
  arc A535 (-24.588, 94.2261) -> (-25.8193, 93.8962) centre (0, 0) ccw
  arc A536 (-22.4914, 91.054) -> (-24.588, 94.2261) centre (-42.797, 79.9125) ccw
  arc A537 (-21.2976, 91.3406) -> (-22.4914, 91.054) centre (0, 0) ccw
  arc A538 (-20.8697, 95.1188) -> (-21.2976, 91.3406) centre (1.8529, 90.632) ccw
  arc A539 (-19.6229, 95.3839) -> (-20.8697, 95.1188) centre (0, 0) ccw
  arc A540 (-17.6952, 92.1063) -> (-19.6229, 95.3839) centre (-38.5561, 82.0428) ccw
  arc A541 (-16.4881, 92.33) -> (-17.6952, 92.1063) centre (0, 0) ccw
  arc A542 (-15.863, 96.0807) -> (-16.4881, 92.33) centre (6.5937, 90.4108) ccw
  arc A543 (-14.604, 96.2801) -> (-15.863, 96.0807) centre (0, 0) ccw
  arc A544 (-12.8505, 92.9062) -> (-14.604, 96.2801) centre (-34.2094, 83.9482) ccw
  arc A545 (-11.6333, 93.0664) -> (-12.8505, 92.9062) centre (0, 0) ccw
  arc A546 (-10.8128, 96.7792) -> (-11.6333, 93.0664) centre (11.3164, 89.9418) ccw
  arc A547 (-9.545, 96.9125) -> (-10.8128, 96.7792) centre (0, 0) ccw
  arc A548 (-7.9705, 93.4514) -> (-9.545, 96.9125) centre (-29.769, 85.6236) ccw
  arc A549 (-6.7466, 93.5477) -> (-7.9705, 93.4514) centre (0, 0) ccw
  arc A550 (-5.7329, 97.2125) -> (-6.7466, 93.5477) centre (16.0081, 89.2263) ccw
  arc A551 (-4.46, 97.2792) -> (-5.7329, 97.2125) centre (0, 0) ccw
  arc A552 (-3.0687, 93.7404) -> (-4.46, 97.2792) centre (-25.2471, 87.0642) ccw
  arc A553 (-1.8415, 93.7726) -> (-3.0687, 93.7404) centre (0, 0) ccw
  arc A554 (-0.6374, 97.3793) -> (-1.8415, 93.7726) centre (20.6559, 88.2662) ccw
  arc A555 (0.6374, 97.3793) -> (-0.6374, 97.3793) centre (0, 0) ccw
  arc A556 (1.8415, 93.7726) -> (0.6374, 97.3793) centre (-20.6559, 88.2662) ccw
  arc A557 (3.0687, 93.7404) -> (1.8415, 93.7726) centre (0, 0) ccw
  arc A558 (4.46, 97.2792) -> (3.0687, 93.7404) centre (25.2471, 87.0642) ccw
  arc A559 (5.7329, 97.2125) -> (4.46, 97.2792) centre (0, 0) ccw
  arc A560 (6.7466, 93.5477) -> (5.7329, 97.2125) centre (-16.0081, 89.2263) ccw
  arc A561 (7.9705, 93.4514) -> (6.7466, 93.5477) centre (0, 0) ccw
  arc A562 (9.545, 96.9125) -> (7.9705, 93.4514) centre (29.769, 85.6236) ccw
  arc A563 (10.8128, 96.7792) -> (9.545, 96.9125) centre (0, 0) ccw
  arc A564 (11.6333, 93.0664) -> (10.8128, 96.7792) centre (-11.3164, 89.9418) ccw
  arc A565 (12.8505, 92.9062) -> (11.6333, 93.0664) centre (0, 0) ccw
  arc A566 (14.604, 96.2801) -> (12.8505, 92.9062) centre (34.2094, 83.9482) ccw
  arc A567 (15.863, 96.0807) -> (14.604, 96.2801) centre (0, 0) ccw
  arc A568 (16.4881, 92.33) -> (15.863, 96.0807) centre (-6.5937, 90.4108) ccw
  arc A569 (17.6952, 92.1063) -> (16.4881, 92.33) centre (0, 0) ccw
  arc A570 (19.6229, 95.3839) -> (17.6952, 92.1063) centre (38.5561, 82.0428) ccw
  arc A571 (20.8697, 95.1188) -> (19.6229, 95.3839) centre (0, 0) ccw
  arc A572 (21.2976, 91.3406) -> (20.8697, 95.1188) centre (-1.8529, 90.632) ccw
  arc A573 (22.4914, 91.054) -> (21.2976, 91.3406) centre (0, 0) ccw
  arc A574 (24.588, 94.2261) -> (22.4914, 91.054) centre (42.797, 79.9125) ccw
  arc A575 (25.8193, 93.8962) -> (24.588, 94.2261) centre (0, 0) ccw
  arc A576 (26.0488, 90.1008) -> (25.8193, 93.8962) centre (2.8929, 90.6048) ccw
  arc A577 (27.226, 89.7521) -> (26.0488, 90.1008) centre (0, 0) ccw
  arc A578 (29.4857, 92.8102) -> (27.226, 89.7521) centre (46.9207, 77.5632) ccw
  arc A579 (30.698, 92.4163) -> (29.4857, 92.8102) centre (0, 0) ccw
  arc A580 (30.7287, 88.614) -> (30.698, 92.4163) centre (7.6309, 90.3292) ccw
  arc A581 (31.8859, 88.2042) -> (30.7287, 88.614) centre (0, 0) ccw
  arc A582 (34.3026, 91.1398) -> (31.8859, 88.2042) centre (50.9157, 75.0012) ccw
  arc A583 (35.4926, 90.683) -> (34.3026, 91.1398) centre (0, 0) ccw
  arc A584 (35.3242, 86.8843) -> (35.4926, 90.683) centre (12.3479, 89.806) ccw
  arc A585 (36.4585, 86.4145) -> (35.3242, 86.8843) centre (0, 0) ccw
  arc A586 (39.0255, 89.2197) -> (36.4585, 86.4145) centre (54.7712, 72.2337) ccw
  arc A587 (40.19, 88.7012) -> (39.0255, 89.2197) centre (0, 0) ccw
  arc A588 (39.823, 84.9165) -> (40.19, 88.7012) centre (17.031, 89.0367) ccw
  arc A589 (40.9311, 84.388) -> (39.823, 84.9165) centre (0, 0) ccw
  arc A590 (43.6414, 87.055) -> (40.9311, 84.388) centre (58.4765, 69.2682) ccw
  arc A591 (44.7772, 86.4762) -> (43.6414, 87.055) centre (0, 0) ccw